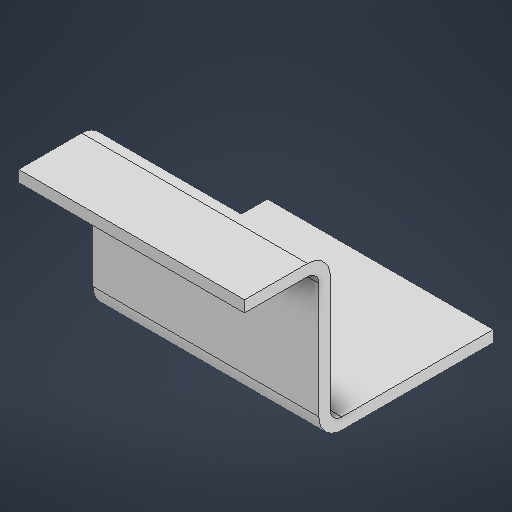
# Autodesk Inventor part: top front joint housing
Saved by Autodesk Inventor 2026.3 (Build 303398000, 398)
## iProperties
Created: 2026-08-05
Part Number: top front joint housing
Material: Generic
Document SubType Name: Sheet Metal
Designer: matot
Density: 1 g/cm^3
Sheet Metal Rule: Default_mm
Appearance: Default
Author: matot
Autodesk Inventor part; units mm, degrees
ref_plane "YZ Plane" through (0, 0, 0) normal (1, 0, 0) x (0, 1, 0)
ref_plane "XZ Plane" through (0, 0, 0) normal (0, 1, 0) x (-1, 0, 0)
ref_plane "XY Plane" through (0, 0, 0) normal (0, 0, 1) x (1, 0, 0)
sketch "Sketch1" plane through (0, 0, 0) normal (0, 1, 0) x (-1, 0, 0)
  line L0 (171.8333, 340.8333) -> (-39.1667, 340.8333)
  line L1 (-39.1667, 340.8333) -> (-39.1667, -59.1667)
  line L2 (-39.1667, -59.1667) -> (171.8333, -59.1667)
  line L3 (171.8333, -59.1667) -> (171.8333, 340.8333)
  point P0 (0, 0)
  dimension "d0" = 400
  dimension "d1" = 211
  measures "d0" distance of L0.end L1.end
  measures "d1" distance of L1.end L2.end
extrude "Plate1" add sketch "Sketch1" along normal blind 4
sketch "Sketch2" plane through (0, 4, 0) normal (0, 1, 0) x (1, 0, 0)
  line L0 (-171.8333, 59.1667) -> (-171.8333, -340.8333) projected
  line L1 (-171.8333, -137.1069) -> (39.1667, -137.1069)
  line L2 (-171.8333, -37.1069) -> (39.1667, -37.1069)
  line L3 (39.1667, -37.1069) -> (39.1667, -37.1069)
  line L4 (39.1667, 59.1667) -> (39.1667, -340.8333) projected
  point P0 (0, 0)
  dimension "d3" = 100
  dimension "d4" = 211
  dimension "d5" = 211
  constraints: 6 end point, 3 perpendicular, 2 point on line, 1 horizontal
  measures "d3" distance between parallel lines of L2 L1
  measures "d4" distance of L2.start L2.end
  measures "d5" distance of L1.start L1.end
fold "Fold1" angle 90 bend radius 4 thickness 4 k factor 0.44 line from (-171.8333, 4, 37.1069) to (39.1667, 4, 37.1069) line at bend centre moving side (0, 0, -1) folds toward (0, 1, 0)
sketch "Sketch3" plane through (0, 0, 0) normal (0, -1, 0) x (1, 0, 0)
  line L0 (39.1667, 41.6308) -> (39.1667, 340.8333) projected
  line L1 (39.1667, 86.6308) -> (-171.8333, 86.6308)
  line L2 (39.1667, 33.6308) -> (-171.8333, 33.6308) projected
  point P0 (0, 0)
  dimension "d12" = 211
  dimension "d13" = 53
  constraints: 2 end point, 1 horizontal, 1 point on line
  measures "d12" distance of L1.start L1.end
  measures "d13" distance between parallel lines of L2 L1
fold "Fold2" angle 90 bend radius 4 thickness 4 k factor 0.44 line from (39.1667, 0, 86.6308) to (-171.8333, 0, 86.6308) line at bend centre moving side (0, 0, -1) folds toward (0, -1, 0)
sketch "Sketch4" plane through (0, 4, 0) normal (0, 1, 0) x (1, 0, 0)
  line L0 (-171.8333, -340.8333) -> (-171.8333, -91.1547) projected
  line L1 (-171.8333, -113.1547) -> (39.1667, -113.1547)
  line L2 (-171.8333, -83.1547) -> (39.1667, -83.1547) projected
  line L3 (39.1667, -91.1547) -> (39.1667, -340.8333) projected
  line L4 (39.1667, -113.1547) -> (-171.8333, -113.1547)
  line L5 (-171.8333, -113.1547) -> (-171.8333, -340.8333)
  line L6 (-171.8333, -340.8333) -> (39.1667, -340.8333)
  line L7 (39.1667, -340.8333) -> (39.1667, -113.1547)
  point P0 (0, 0)
  point P1 (-66.3333, -83.1547)
  dimension "d20" = 211
  dimension "d21" = 30
  constraints: 10 end point, 2 horizontal, 2 parallel, 2 perpendicular, 1 midpoint, 1 point on line
  measures "d20" distance of L1.start L1.end
  measures "d21" distance from line of point (-66.333, -83.155) L1
extrude "Cut1" cut sketch "Sketch4" against normal through all
sketch "Sketch5" plane through (-171.8333, -52.4761, -12.595) normal (0, -1, 0) x (1, 0, 0)
  line L0 (0, 0) -> (0, 91.7497) projected
  line L1 (0, 38.7497) -> (211, 38.7497)
  line L2 (0, 99.7497) -> (211, 99.7497) projected
  line L3 (211, 91.7497) -> (211, 0) projected
  line L4 (211, 0) -> (0, 0) projected
  line L5 (211, 38.7497) -> (0, 38.7497)
  line L6 (0, 38.7497) -> (0, 0)
  line L7 (0, 0) -> (211, 0)
  line L8 (211, 0) -> (211, 38.7497)
  point P0 (171.8333, 12.595)
  dimension "d24" = 211
  dimension "d25" = 61
  constraints: 10 end point, 2 horizontal, 2 parallel, 2 perpendicular, 1 point on line
  measures "d24" distance of L1.start L1.end
  measures "d25" distance between parallel lines of L2 L1
extrude "Cut2" cut sketch "Sketch5" against normal through all
sketch "Sketch6" plane through (-171.8333, -44.4761, 87.1547) normal (0, 0, 1) x (1, 0, 0)
  line L0 (211, 48.4761) -> (0, 48.4761) projected
  line L1 (211, -8) -> (0, -8) projected
  line L2 (89, 48.4761) -> (129, 48.4761)
  line L3 (129, 48.4761) -> (129, -8)
  line L4 (129, -8) -> (89, -8)
  line L5 (89, -8) -> (89, 48.4761)
  line L6 (0, 0) -> (0, 40.4761) projected
  line L7 (89, -8) -> (129, -8)
  line L8 (129, -8) -> (129, 48.4761)
  line L9 (129, 48.4761) -> (89, 48.4761)
  line L10 (89, 48.4761) -> (89, -8)
  point P0 (171.8333, 44.4761)
  point P1 (129, 20.2381)
  point P2 (89, 20.2381)
  point P3 (89, -8)
  point P4 (129, 48.4761)
  dimension "d28" = 40
  dimension "d29" = 89
  constraints: 16 end point, 4 parallel, 2 horizontal, 2 midpoint, 2 perpendicular, 2 point on line
  measures "d28" distance of point (129, 20.238) point (89, 20.238)
  measures "d29" distance between parallel lines of L6 L5
extrude "Cut3" cut sketch "Sketch6" along normal through all
sketch "Sketch7" plane through (-171.8333, -44.4761, 87.1547) normal (0, 0, 1) x (1, 0, 0)
  line L0 (89, 48.4761) -> (0, 48.4761) projected
  line L1 (211, -8) -> (0, -8) projected
  line L2 (89, 48.4761) -> (129, 48.4761)
  line L3 (129, 48.4761) -> (129, -8)
  line L4 (129, -8) -> (89, -8)
  line L5 (89, -8) -> (89, 48.4761)
  point P0 (171.8333, 44.4761)
  point P1 (89, -8)
  constraints: 8 end point, 2 parallel, 1 horizontal, 1 perpendicular, 1 point on line
extrude "Cut4" cut sketch "Sketch7" against normal through all
sketch "Sketch8" plane through (-42.8333, -44.4761, 87.1547) normal (-1, 0, 0) x (0, 0, 1)
  line L0 (0, -8) -> (-4, -8)
  line L1 (-4, -4) -> (-4, 48.4761)
  line L2 (-4, 48.4761) -> (0, 48.4761)
  line L3 (0, 44.4761) -> (0, -8)
  line L4 (4, 44.4761) -> (26, 44.4761) projected
  line L5 (26, 44.4761) -> (0, 44.4761)
  line L6 (-4, 53.4761) -> (-4, 48.4761)
  line L7 (-4, 48.4761) -> (26, 48.4761)
  line L8 (26, 48.4761) -> (26, 44.4761)
  line L9 (-61, -8) -> (0, -8)
  line L10 (0, -8) -> (0, -4)
  line L11 (-4, -4) -> (-61, -4)
  line L12 (-61, -4) -> (-61, -8)
  point P0 (-87.1547, 44.4761)
  point P1 (0, 48.4761)
  point P2 (-4, -8)
  dimension "d34" = 4
  dimension "d35" = 4
  constraints: 24 end point, 6 parallel, 3 horizontal, 3 perpendicular, 1 point on line
  measures "d34" distance between parallel lines of L4 L7
  measures "d35" distance between parallel lines of L9 L11
extrude "Cut5" cut sketch "Sketch8" against normal through all
sketch "Sketch9" plane through (-42.8333, -4, 87.1547) normal (-1, 0, 0) x (0, 0, 1)
  arc A0 (4, 4) -> (0, 0) centre (4, 0) ccw projected
  line L0 (0, 0) -> (4, 0)
  line L1 (4, 0) -> (4, 4)
  line L2 (4, 4) -> (0, 4)
  line L3 (0, 4) -> (0, 0)
  arc A1 (-8, -44.4761) -> (-4, -40.4761) centre (-8, -40.4761) ccw projected
  line L4 (-4, -40.4761) -> (-8, -40.4761)
  line L5 (-8, -40.4761) -> (-8, -44.4761)
  line L6 (-8, -44.4761) -> (-4, -44.4761)
  line L7 (-4, -44.4761) -> (-4, -40.4761)
  point P0 (-87.1547, 4)
  constraints: 16 end point, 4 parallel, 2 horizontal, 2 perpendicular, 1 point on circle
extrude "Cut6" cut sketch "Sketch9" against normal through all
sketch "Sketch10" plane through (-82.8333, -44.4761, 87.1547) normal (1, 0, 0) x (0, 0, -1)
  line L0 (-28, 44.4761) -> (-4, 44.4761)
  line L1 (4, 44.4761) -> (4, 50.4761)
  line L2 (4, 50.4761) -> (-28, 50.4761)
  line L3 (-28, 50.4761) -> (-28, 44.4761)
  line L4 (0, -8) -> (4, -8)
  line L5 (4, 0) -> (4, 50.4761)
  line L6 (4, 50.4761) -> (0, 50.4761)
  line L7 (0, 40.4761) -> (0, -8)
  line L8 (61, -4) -> (8, -4)
  line L9 (0, -4) -> (0, -8)
  line L10 (0, -8) -> (61, -8)
  line L11 (61, -8) -> (61, -4)
  arc A0 (0, 40.4761) -> (-4, 44.4761) centre (-4, 40.4761) ccw
  line L12 (-4, 44.4761) -> (-26, 44.4761) projected
  arc A1 (4, 0) -> (8, -4) centre (8, 0) ccw
  point P0 (87.1547, 44.4761)
  point P1 (4, -8)
  point P2 (4, 44.4761)
  dimension "d40" = 4
  dimension "d41" = 0
  dimension "d42" = 4
  constraints: 24 end point, 6 parallel, 4 point on circle, 4 point on line, 4 tangent, 3 horizontal, 3 perpendicular, 2 centre point
  measures "d40" radius of A0
  measures "d41" distance between parallel lines of L12 L0
  measures "d42" radius of A1
extrude "Cut7" cut sketch "Sketch10" against normal blind 10
equation "\"d2\" = Thickness"
equation "\"d6\" = BendReliefWidth"
equation "\"d7\" = BendReliefDepth"
equation "\"d8\" = MinimumRemnant"
equation "\"d9\" = TransitionRadius"
equation "\"d11\" = BendRadius"
equation "\"d14\" = BendReliefWidth"
equation "\"d15\" = BendReliefDepth"
equation "\"d16\" = MinimumRemnant"
equation "\"d17\" = TransitionRadius"
equation "\"d19\" = BendRadius"
equation "\"d22\" = Thickness"
equation "\"d26\" = Thickness"
equation "\"d30\" = Thickness"
equation "\"d32\" = Thickness"
equation "\"d36\" = Thickness"
equation "\"d38\" = Thickness"
equation "\"BendRadius\" = Thickness"
equation "\"BendReliefWidth\" = Thickness"
equation "\"BendReliefDepth\" = 0.5 * Thickness"
equation "\"CornerReliefSize\" = 4 * Thickness"
equation "\"MinimumRemnant\" = 2 * Thickness"
equation "\"TransitionRadius\" = BendRadius"
equation "\"JacobiRadiusSize\" = BendRadius"
equation "\"GapSize\" = Thickness"
equation "\"Thickness\" = 4"
body "Solid1"
